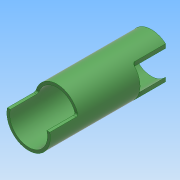
# Autodesk Inventor part: Pancake_Drop Pipe
Saved by Autodesk Inventor 2018.1 (Build 221171000, 171)
## iProperties
Created: 2019-02-21
Part Number: Pancake_Drop Pipe
Material: PVC-Piping
Document SubType Name: Modeling
Designer: James
Density: 1.4 g/cm^3
Appearance: Smooth - Dark Forest Green
Author: James
Autodesk Inventor part; units mm, degrees
ref_plane "YZ Plane" through (0, 0, 0) normal (1, 0, 0) x (0, 1, 0)
ref_plane "XZ Plane" through (0, 0, 0) normal (0, 1, 0) x (-1, 0, 0)
sketch "Sketch1" plane through (0, 0, 0) normal (0, 1, 0) x (-1, 0, 0)
  circle A0 centre (0, 0) radius 20
  circle A1 centre (0, 0) radius 23
  dimension "d0" = 40
  dimension "d1" = 3
  constraints: 2 centre point, 2 coincident
  measures "d0" diameter of A0
  measures "d1" radial gap between concentric circles of A0 A1
extrude "Extrusion1" add sketch "Sketch1" along normal blind 130
ref_plane "Work Plane1" through (0, 0, 23) normal (0, 0, 1) x (1, 0, 0)
sketch "Sketch2" plane through (0, 0, 23) normal (0, 0, 1) x (1, 0, 0)
  line L0 (-17.5, 120) -> (17.5, 120)
  line L1 (17.5, 120) -> (17.5, 85)
  line L2 (17.5, 85) -> (-17.5, 85)
  line L3 (-17.5, 85) -> (-17.5, 120)
  line L4 (-17.5, 70) -> (17.5, 70)
  line L5 (17.5, 70) -> (17.5, 35)
  line L6 (17.5, 35) -> (-17.5, 35)
  line L7 (-17.5, 35) -> (-17.5, 70)
  line L8 (23, 130) -> (-23, 130) projected
  line L9 (0, 162) -> (0, -27) projected
  line L10 (-23, 0) -> (23, 0) projected
  point P0 (0, 0)
  dimension "d5" = 10
  dimension "d6" = 35
  dimension "d7" = 17.5
  dimension "d8" = 35
  dimension "d9" = 35
  dimension "d23" = 15
  dimension "d24" = 35
  constraints: 16 end point, 4 parallel, 2 horizontal, 2 perpendicular, 2 vertical alignment
  measures "d5" distance between parallel lines of L8 L0
  measures "d6" distance of L0.start L0.end
  measures "d7" distance between parallel lines of L1 L9
  measures "d8" distance of L0.end L1.end
  measures "d9" distance of L4.end L5.end
  measures "d23" distance between parallel lines of L4 L2
  measures "d24" distance between parallel lines of L10 L6
extrude "Extrusion2" [suppressed]
fillet "Fillet1" [suppressed]
sketch "Sketch3" plane through (0, 0, 0) normal (0, 0, 1) x (1, 0, 0)
  line L0 (23, 130) -> (-23, 130) projected
  point P0 (0, 0)
  point P1 (0, 80)
  point P2 (0, 50)
  dimension "d14" = 30
  dimension "d15" = 50
  constraints: 2 vertical alignment
  measures "d14" distance of point (0, 50) point (0, 80)
  measures "d15" distance from line of point (0, 80) L0
hole "Hole1" at (0, 80, 0) at (0, 50, 0) direction (0, 0, -1) diameter 4.5 end through all clearance for "Socket Head Cap Screw" size "M4" standard "Ansi Metric M Profile"
sketch "Sketch4" plane through (0, 130, 0) normal (0, 1, 0) x (1, 0, 0)
  circle A0 centre (0, 0) radius 20 projected
  circle A1 centre (0, 0) radius 23 projected
  line L0 (15, 17.4356) -> (15, -17.4356)
  circle A2 centre (0, 0) radius 23 projected
  dimension "d25" = 15
  constraints: 2 end point, 1 point on circle, 1 vertical, 2 other
  measures "d25" distance from line of L0 point (0, 0)
extrude "Extrusion3" cut sketch "Sketch4" against normal blind 35 contours A0 L0 | A0 L0 A1 picked at (16.6667, 0) picked at (17.0329, 12.1097)
fillet "Fillet2" radius 2 2 edges at (15, 95, -15.3322) (15, 95, 15.3322)
sketch "Sketch5" plane through (0, 0, 0) normal (0, -1, 0) x (1, 0, 0)
  circle A0 centre (0, 0) radius 20 projected
  circle A1 centre (0, 0) radius 23 projected
  line L0 (-22.4499, 5) -> (22.4499, 5)
  circle A2 centre (0, 0) radius 23 projected
  dimension "d29" = 5
  constraints: 2 end point, 1 horizontal, 1 point on circle, 2 other
  measures "d29" distance from line of L0 point (0, 0)
extrude "Extrusion4" cut sketch "Sketch5" against normal blind 30 contours L0 A0 | A0 L0 A1 picked at (5.8749, 6.4846) picked at (-0.7969, 21.8366)
fillet "Fillet3" radius 2 2 edges at (-20.9074, 30, 5) (20.9074, 30, 5)
equation "\"d7\" = 0.5 * d6"
equation "\"d8\" = d6"
equation "\"d9\" = d8"
body "Solid1"
